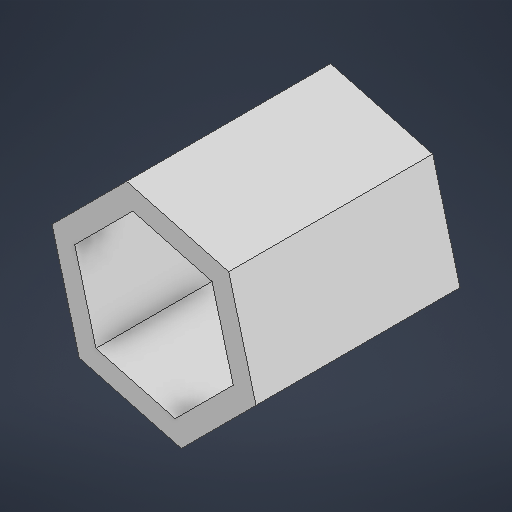
# Autodesk Inventor part: Part2
Saved by Autodesk Inventor 2026.2 (Build 302298010, 298A)
## iProperties
Created: 2026-04-16
Part Number: Part2
Material: Generic
Document SubType Name: Modeling
Designer: mrcm
Density: 1 g/cm^3
Appearance: Default
Author: mrcm
Autodesk Inventor part; units mm, degrees
ref_plane "YZ Plane" through (0, 0, 0) normal (1, 0, 0) x (0, 1, 0)
ref_plane "XZ Plane" through (0, 0, 0) normal (0, 1, 0) x (-1, 0, 0)
ref_plane "XY Plane" through (0, 0, 0) normal (0, 0, 1) x (1, 0, 0)
sketch "Sketch1" plane through (0, 0, 0) normal (0, 0, 1) x (1, 0, 0)
  line L0 (-2.6795, 10) -> (7.3205, 7.3205)
  line L1 (7.3205, 7.3205) -> (10, -2.6795)
  line L2 (10, -2.6795) -> (2.6795, -10)
  line L3 (2.6795, -10) -> (-7.3205, -7.3205)
  line L4 (-7.3205, -7.3205) -> (-10, 2.6795)
  line L5 (-10, 2.6795) -> (-2.6795, 10)
  point P0 (0, 0)
  point P1 (0, 0)
  dimension "d0" = 10
  dimension "d2" = 10
  constraints: 12 end point, 1 coincident, 13 other
  measures "d0" horizontal distance of L0.start L0.end
  measures "d2" vertical distance of L0.end L1.end
extrude "Extrusion1" add sketch "Sketch1" along normal blind 20
shell "Shell1" thickness 2 removed faces 1 at (-3.3333, 0.8932, 20)
shell "Shell2" thickness 2 removed faces 8 at (-3.3333, 0.8932, 0) at (-5.8735, 3.9776, 14) at (0.508, 7.0754, 8) at (6.3814, 3.0978, 14) at (5.8735, -3.9776, 14) at (-0.508, -7.0754, 14) at (-7.0754, -0.508, 8) at (1.8958, 1.8958, 2)
body "Solid1"
